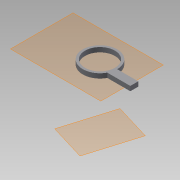
# Autodesk Inventor part: 15_Gabel
Saved by Autodesk Inventor 2015 (Build 190159000, 159)
## iProperties
Created: 2016-03-16
Part Number: 15_Gabel
Material: Generisch
Document SubType Name: Modeling
Designer: Bene
Density: 1 g/cm^3
Appearance: Vorgabe
Author: Bene
Autodesk Inventor part; units mm, degrees
ref_plane "YZ Plane" through (0, 0, 0) normal (1, 0, 0) x (0, 1, 0)
ref_plane "XZ Plane" through (0, 0, 0) normal (0, 1, 0) x (-1, 0, 0)
ref_plane "XY Plane" through (0, 0, 0) normal (0, 0, 1) x (1, 0, 0)
ref_plane "Arbeitsebene1" through (-1.9028, 0, 2) normal (0, 0, 1) x (-0.2882, -0.9576, 0)
sketch "Skizze1" plane through (-1.9028, 0, 2) normal (0, 0, 1) x (-0.2882, -0.9576, 0)
  circle A0 centre (-14.632, 0) radius 18.75
  circle A1 centre (-14.632, 0) radius 15
  circle A2 centre (-14.632, 0) radius 16.2815
  line L0 (26.7708, -9) -> (26.7708, -29)
  line L1 (19.0208, -9) -> (26.7708, -9)
  line L2 (26.7708, -29) -> (19.0208, -29)
  line L3 (27.1135, -8.6759) -> (1.6495, -8.6759)
  line L4 (1.6495, -8.6759) -> (1.6495, 0)
  line L5 (1.6495, 0) -> (27.1135, 0)
  line L6 (27.1135, 0) -> (27.1135, -8.6759)
  point P0 (-12.7292, 0)
  constraints: 14 end point, 2 centre point, 2 parallel, 1 horizontal, 1 horizontal alignment, 1 perpendicular, 2 other
extrude "Extrusion1" add sketch "Skizze1" along normal blind 5 contours L5 L4 L3 A0 | L5 L6 L3 A0 | A0 L3 L4 L5
